Test (Autodesk Fusion 360 design; units mm, degrees)
Autodesk Fusion 360 part; units mm, degrees
sketch "Sketch1" plane through (0, 0, 0) normal (0, 0, 1) x (1, 0, 0)
  line L0 (27.6067, 32.2429) -> (-27.6067, 32.2429)
  line L1 (-27.6067, 32.2429) -> (-27.6067, -32.2429)
  line L2 (-27.6067, -32.2429) -> (27.6067, -32.2429)
  line L3 (27.6067, -32.2429) -> (27.6067, 32.2429)
  line L4 (27.6067, 32.2429) -> (-27.6067, -32.2429) construction
  line L5 (-27.6067, 32.2429) -> (27.6067, -32.2429) construction
  constraint horizontal L0
  constraint perpendicular L0 L1
  constraint parallel L0 L2
  constraint parallel L1 L3
  constraint coincident L4 origin
  constraint coincident L5 origin
extrude "Extrude1" add sketch "Sketch1" along normal blind 20
sketch "Sketch2" plane through (0, 0, 20) normal (0, 0, 1) x (-1, 0, 0)
  line L0 (-27.6067, 32.2429) -> (-27.6067, -32.2429)
  line L1 (-27.6067, -32.2429) -> (27.6067, -32.2429)
  line L2 (27.6067, -32.2429) -> (27.6067, 32.2429)
  line L3 (27.6067, 32.2429) -> (-27.6067, 32.2429)
  circle A0 centre (0, 0) radius 11.8335
  constraint coincident A0.centre origin
extrude "Extrude2" add sketch "Sketch2" along normal blind 20 contours A0
sketch "Sketch4" plane through (0, -32.2429, 0) normal (0, -1, 0) x (1, 0, 0)
  line L0 (-27.6067, 0) -> (27.6067, 0)
  line L1 (27.6067, 0) -> (27.6067, 20)
  line L2 (27.6067, 20) -> (-27.6067, 20)
  line L3 (-27.6067, 20) -> (-27.6067, 0)
  line L4 (-7.3118, 13.4579) -> (10.9147, 11.7624)
  line L5 (10.9147, 11.7624) -> (10.2462, 4.5769)
  line L6 (10.2462, 4.5769) -> (-7.9802, 6.2724)
  line L7 (-7.9802, 6.2724) -> (-7.3118, 13.4579)
  constraint perpendicular L4 L5
  constraint parallel L4 L6
  constraint parallel L5 L7
extrude "Extrude4" add sketch "Sketch4" along normal blind 10 contours L4 L5 L6 L7
sketch "Sketch3" plane through (0, 0, 40) normal (0, 0, 1) x (-1, 0, 0)
  circle A0 centre (0, 0) radius 11.8335
  circle A1 centre (0, 0) radius 4.7343
  constraint concentric A0 A1
extrude "Extrude3" [suppressed]
